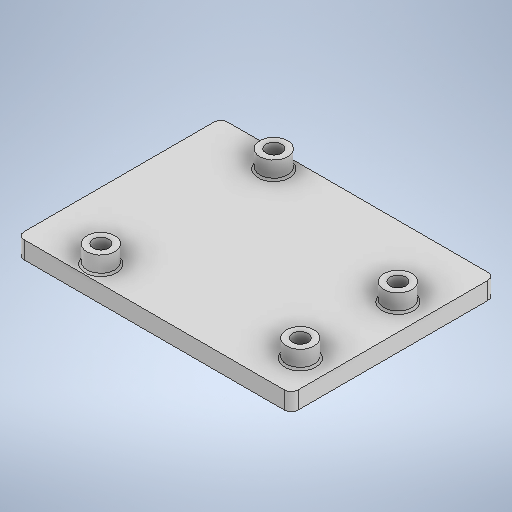
# Autodesk Inventor part: Leonardo_Backplate
Saved by Autodesk Inventor 2025.2 (Build 292293000, 293)
## iProperties
Created: 2025-04-21
Part Number: Leonardo_Backplate
Material: Generic
Document SubType Name: Modeling
Designer: osmon
Density: 1 g/cm^3
Appearance: Default
Author: osmon
Autodesk Inventor part; units mm, degrees
ref_plane "YZ Plane" through (0, 0, 0) normal (1, 0, 0) x (0, 1, 0)
ref_plane "XZ Plane" through (0, 0, 0) normal (0, 1, 0) x (-1, 0, 0)
ref_plane "XY Plane" through (0, 0, 0) normal (0, 0, 1) x (1, 0, 0)
sketch "Sketch1" plane through (0, 0, 0) normal (0, 1, 0) x (-1, 0, 0)
  line L0 (0, 0) -> (-78.6, 0)
  line L1 (-78.6, 0) -> (-78.6, -58.4)
  line L2 (-78.6, -58.4) -> (0, -58.4)
  line L3 (0, -58.4) -> (0, 0)
  dimension "d0" = 78.6
  dimension "d1" = 58.4
  constraints: 8 end point, 2 parallel, 1 horizontal, 1 perpendicular
  measures "d0" distance of L2.end L1.end
  measures "d1" distance of L1.end L0.end
extrude "Extrusion1" add sketch "Sketch1" along normal blind 5
sketch "Sketch2" plane through (0, 5, 0) normal (0, 1, 0) x (1, 0, 0)
  circle A0 centre (19, 5) radius 4
  line L0 (0, 58.4) -> (0, 0) projected
  line L1 (0, 0) -> (78.6, 0) projected
  circle A1 centre (20.2, 53.4) radius 4
  line L2 (78.6, 58.4) -> (0, 58.4) projected
  circle A2 centre (71, 38.2) radius 4
  circle A3 centre (71, 10.2) radius 4
  line L3 (78.6, 0) -> (78.6, 58.4) projected
  dimension "d4" = 8
  dimension "d5" = 19
  dimension "d6" = 5
  dimension "d7" = 8
  dimension "d8" = 20.2
  dimension "d9" = 5
  dimension "d10" = 8
  dimension "d11" = 8
  dimension "d12" = 20.2
  dimension "d13" = 7.6
  dimension "d14" = 7.6
  dimension "d15" = 28
  constraints: 4 centre point
  measures "d4" diameter of A0
  measures "d5" distance from line of L0 A0.centre
  measures "d6" distance from line of L1 A0.centre
  measures "d7" diameter of A1
  measures "d8" distance from line of L0 A1.centre
  measures "d9" distance from line of L2 A1.centre
  measures "d10" diameter of A2
  measures "d11" diameter of A3
  measures "d12" distance from line of L2 A2.centre
  measures "d13" distance from line of L3 A2.centre
  measures "d14" distance from line of L3 A3.centre
  measures "d15" distance of A3.centre A2.centre
extrude "Extrusion2" add sketch "Sketch2" along normal blind 5 contours A0 | A1 | A2 | A3
sketch "Sketch3" plane through (20.2, 10, -53.4) normal (0, 1, 0) x (1, 0, 0)
  circle A0 centre (50.8, -15.2) radius 4 projected
  circle A1 centre (0, 0) radius 4 projected
  circle A2 centre (-1.2, -48.4) radius 4 projected
  circle A3 centre (50.8, -43.2) radius 4 projected
  circle A4 centre (0, 0) radius 2.25
  circle A5 centre (50.8, -15.2) radius 2.25
  circle A6 centre (-1.2, -48.4) radius 2.25
  circle A7 centre (50.8, -43.2) radius 2.25
  point P0 (-20.2, -53.4)
  dimension "d18" = 4.5
  dimension "d19" = 4.5
  dimension "d20" = 4.5
  dimension "d21" = 4.5
  constraints: 4 centre point, 4 coincident
  measures "d18" diameter of A4
  measures "d19" diameter of A5
  measures "d20" diameter of A6
  measures "d21" diameter of A7
extrude "Extrusion3" cut sketch "Sketch3" against normal blind 4.2 contours A4 | A5 | A6 | A7
sketch "Sketch4" plane through (20.2, 5.8, -53.4) normal (0, 1, 0) x (1, 0, 0)
  circle A0 centre (0, 0) radius 2.25 projected
  circle A1 centre (50.8, -15.2) radius 2.25 projected
  circle A2 centre (50.8, -43.2) radius 2.25 projected
  circle A3 centre (-1.2, -48.4) radius 2.25 projected
  circle A4 centre (0, 0) radius 1.6
  circle A5 centre (50.8, -15.2) radius 1.6
  circle A6 centre (50.8, -43.2) radius 1.6
  circle A7 centre (-1.2, -48.4) radius 1.6
  point P0 (-20.2, -53.4)
  dimension "d24" = 3.2
  dimension "d25" = 3.2
  dimension "d26" = 3.2
  dimension "d27" = 3.2
  constraints: 4 centre point, 4 coincident
  measures "d24" diameter of A4
  measures "d25" diameter of A5
  measures "d26" diameter of A6
  measures "d27" diameter of A7
extrude "Extrusion4" cut sketch "Sketch4" against normal blind 2 contours A4 | A5 | A6 | A7
chamfer "Chamfer1" distance 0.5 angle 45 4 edges at (16.2, 5, -53.4) (15, 5, -5) (67, 5, -10.2) (67, 5, -38.2)
fillet "Fillet1" radius 2 4 edges at (0, 2.5, -58.4) (0, 2.5, 0) (78.6, 2.5, 0) (78.6, 2.5, -58.4)
body "Solid1"
